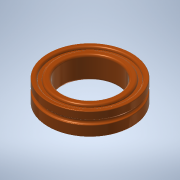
# Autodesk Inventor part: ROLAMENTO_INFERIOR_INTERNO
Saved by Autodesk Inventor 2020.4 (Build 244396000, 396)
## iProperties
Created: 2016-03-03
Part Number: ROLAMENTO_INFERIOR_INTERNO
Material: Genérico
Document SubType Name: Modeling
Designer: Everton
Density: 1 g/cm^3
Appearance: Padrão
Author: Everton
Autodesk Inventor part; units mm, degrees
ref_plane "YZ Plane" through (0, 0, 0) normal (1, 0, 0) x (0, 1, 0)
ref_plane "XZ Plane" through (0, 0, 0) normal (0, 1, 0) x (-1, 0, 0)
ref_plane "XY Plane" through (0, 0, 0) normal (0, 0, 1) x (1, 0, 0)
sketch "Sketch1" plane through (0, 0, 0) normal (0, 1, 0) x (-1, 0, 0)
  line L0 (1.5806, 18.0935) -> (58.0806, 18.0935)
  line L1 (58.0806, 18.0935) -> (58.0806, 8.0935)
  line L2 (58.0806, 2.0935) -> (58.0806, -11.9065)
  line L3 (58.0806, -11.9065) -> (1.5806, -11.9065)
  line L4 (1.5806, -11.9065) -> (1.5806, 18.0935)
  arc A0 (58.0806, 8.0935) -> (58.0806, 2.0935) centre (58.0806, 5.0935) ccw
  point P0 (0, 0)
  dimension "d0" = 56.5
  dimension "d1" = 10
  dimension "d39" = 6
  dimension "d40" = 17
  constraints: 10 end point, 3 perpendicular, 2 point on circle, 1 centre point, 1 horizontal, 1 point on line, 1 vertical
  measures "d0" distance of L0.start L0.end
  measures "d1" distance of L0.end L1.end
  measures "d39" diameter of A0
  measures "d40" distance of L2.end A0.centre
revolve "Revolution1" add sketch "Sketch1" angle 360 about axis through (-1.5806, 0, -11.9065) along (0, 0, 1)
fillet "Fillet1" radius 1 2 edges at (54.9194, 0, 8.0935) (54.9194, 0, 2.0935)
fillet "Fillet4" radius 1 1 edges at (54.9194, 0, -11.9065)
fillet "Fillet5" radius 1 1 edges at (54.9194, 0, 18.0935)
sketch "Sketch3" plane through (-1.5806, 0, -11.9065) normal (0, 0, -1) x (-1, 0, 0)
  line L0 (1.9194, -50) -> (7.9194, -50)
  line L1 (1.9194, -50) -> (-4.0806, -50)
  line L2 (1.9194, 50) -> (7.9194, 50)
  line L3 (7.9194, 50) -> (-4.0806, 50)
  line L4 (-1.5806, 0) -> (68.9222, 70.5028)
  line L5 (-1.5806, 0) -> (-1.5806, 80.0451)
  line L6 (-1.5806, 0) -> (25.001, 0)
  line L7 (-1.5806, 0) -> (33.7747, 35.3553)
  line L8 (33.7747, 35.3553) -> (38.0174, 31.1127)
  line L9 (38.0174, 31.1127) -> (29.5321, 39.598)
  point P0 (38.0174, -31.1127)
  point P1 (29.5321, -39.598)
  dimension "d21" = 45
  dimension "d22" = 50
  dimension "d23" = 6
  dimension "d24" = 12
  constraints: 20 end point, 3 point on line, 2 coincident, 2 horizontal, 2 symmetric about line, 1 perpendicular, 1 vertical
  measures "d21" angle of L5 L4
  measures "d22" distance of L4.start L7.end
  measures "d23" distance of L7.end L8.end
  measures "d24" distance of L8.end L9.end
hole "Hole1" at (-39.598, 31.1127, -11.9065) at (-31.1127, 39.598, -11.9065) direction (0, 0, 1) diameter 3.242 depth 11.8 tip angle 118 thread size "M4x0.7" class "6H" standard "ISO Metric profile"
sketch "Sketch5" plane through (-1.5806, 0, 18.0935) normal (0, 0, 1) x (1, 0, 0)
  circle A0 centre (0, 0) radius 55.75 projected
  circle A1 centre (0, 0) radius 37
  point P0 (1.5806, 0)
  dimension "d41" = 74
  constraints: 1 centre point, 1 coincident
  measures "d41" diameter of A1
extrude "Extrusion3" cut sketch "Sketch5" against normal blind 300 contours A1
fillet "Fillet9" radius 3 2 edges at (-38.5806, 0, 18.0935) (-38.5806, 0, -11.9065)
sketch "Sketch6" plane through (-1.5806, 0, 18.0935) normal (0, 0, 1) x (1, 0, 0)
  circle A0 centre (0, 0) radius 37 projected
  circle A1 centre (0, 0) radius 50
  circle A2 centre (0, 0) radius 46
  point P0 (1.5806, 0)
  dimension "d45" = 100
  dimension "d46" = 92
  constraints: 2 centre point, 2 coincident
  measures "d45" diameter of A1
  measures "d46" diameter of A2
extrude "Extrusion4" cut sketch "Sketch6" against normal blind 3 contours A1
fillet "Fillet10" radius 3 2 edges at (-51.5806, 0, 18.0935) (-47.5806, 0, 18.0935)
hole "Hole2" at (-31.1127, -39.598, -11.9065) at (-39.598, -31.1127, -11.9065) direction (0, 0, 1) diameter 3.242 depth 11.8 tip angle 118 thread size "M4x0.7" class "6H" standard "ISO Metric profile"
body "Solid1"
